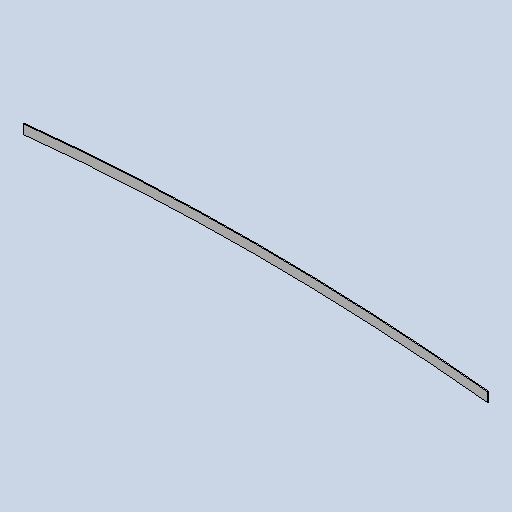
# Autodesk Inventor part: MSC 407 sheet lowerback_FIX
Saved by Autodesk Inventor 2025 (Build 290162010, 162A)
## iProperties
Created: 2024-04-18
Part Number: MSC 407 sheet lowerback_FIX
Material: Stainless Steel AISI 304
Document SubType Name: Sheet Metal
Designer: DELL
Stock Number: МОО 407 лист поясница_фиксированный
Mass: 24644.5 g
Surface Area: 20691.2 cm^2
Volume: 3080.57 cm^3
Density: 8 g/cm^3
Flat Pattern Width: 150 cm
Flat Pattern Length: 6.9169 cm
Flat Pattern Area: 1037.54 cm^2
Sheet Metal Rule: Default_mm
Sheet Metal Width: 1500,000 mm
Sheet Metal Length: 69,169 mm
Sheet Metal Area: 103753,564 mm^2
Appearance: Default
Description: Добавочный лист к пояснице
Поясница_радиус: 8688,266 mm
Author: admin
Autodesk Inventor part; units mm, degrees
ref_plane "YZ Plane" through (0, 0, 0) normal (1, 0, 0) x (0, 1, 0)
ref_plane "XZ Plane" through (0, 0, 0) normal (0, 1, 0) x (-1, 0, 0)
ref_plane "XY Plane" through (0, 0, 0) normal (0, 0, 1) x (1, 0, 0)
sketch "Sketch5" plane through (0, 0, 0) normal (0, 0, 1) x (1, 0, 0)
  arc A0 (750, -39.169) -> (-750, -39.169) centre (0, -7200) ccw
  line L0 (-750, -39.169) -> (-750, -69.169)
  line L1 (750, -39.169) -> (750, -69.169)
  arc A1 (750, -69.169) -> (-750, -69.169) centre (0, -7200) ccw
  point P0 (0, 0)
  point P1 (0, 0)
  dimension "d30" = 7200
  dimension "d31" = 30
  dimension "d32" = 1500
  measures "d30" radius of A0
  measures "d31" distance of L1.start L1.end
  measures "d32" distance between parallel lines of L1 L0
extrude "Plate2" add sketch "Sketch5" along normal blind 3
equation "\"d33\" = Thickness"
equation "\"BendRadius\" = Thickness"
equation "\"BendReliefWidth\" = Thickness"
equation "\"BendReliefDepth\" = 0.5 * Thickness"
equation "\"CornerReliefSize\" = 4 * Thickness"
equation "\"MinimumRemnant\" = 2 * Thickness"
equation "\"TransitionRadius\" = BendRadius"
equation "\"JacobiRadiusSize\" = BendRadius"
equation "\"GapSize\" = Thickness"
equation "\"Поясница_радиус\" = d21"
equation "\"Thickness\" = 3"
equation "\"d21\" = 8688.265625"
body "Solid2"
